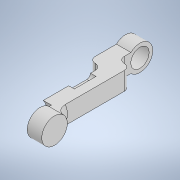
# Autodesk Inventor part: Рулевая тяга
Saved by Autodesk Inventor 2020 (Build 240168000, 168)
## iProperties
Created: 2021-07-18
Part Number: Рулевая тяга
Material: Типовые
Document SubType Name: Modeling
Designer: Антон
Density: 1 g/cm^3
Appearance: По умолчанию
Author: Антон
Autodesk Inventor part; units mm, degrees
ref_plane "YZ Plane" through (0, 0, 0) normal (1, 0, 0) x (0, 1, 0)
ref_plane "XZ Plane" through (0, 0, 0) normal (0, 1, 0) x (-1, 0, 0)
ref_plane "XY Plane" through (0, 0, 0) normal (0, 0, 1) x (1, 0, 0)
sketch "Эскиз1" plane through (0, 0, 0) normal (0, 1, 0) x (-1, 0, 0)
  line L0 (0, 0) -> (4, 0)
  line L1 (4, 0) -> (4, -23.1503)
  line L2 (4, -23.1503) -> (0, -23.1503)
  line L3 (0, -23.1503) -> (0, 0)
  line L4 (0, -23.1503) -> (7.35, -23.1503)
  line L5 (7.35, -23.1503) -> (7.35, -19.1503)
  line L6 (7.35, -19.1503) -> (0, -19.1503)
  line L7 (0, -19.1503) -> (0, -23.1503)
  line L8 (7.35, -19.1503) -> (3.35, -19.1503)
  line L9 (3.35, -19.1503) -> (3.35, -29.1503)
  line L10 (3.35, -29.1503) -> (7.35, -29.1503)
  line L11 (7.35, -29.1503) -> (7.35, -19.1503)
  line L12 (7.35, -23.1503) -> (4, -19.1503)
  line L13 (0, -19.1503) -> (3.35, -23.1503)
  point P0 (4, -19.1503)
  point P1 (0, -19.1503)
  point P2 (4, -19.1503)
  dimension "d10" = 4
  dimension "d11" = 7.35
  dimension "d36" = 29.1503
  dimension "d55" = 10
  constraints: 28 end point, 6 parallel, 4 point on line, 3 horizontal, 3 perpendicular, 2 equal length
  measures "d10" distance of L0.start L0.end
  measures "d11" distance between parallel lines of L3 L11
  measures "d36" distance between parallel lines of L10 L0
  measures "d55" distance of L10.end L5.end
extrude "Выдавливание1" add sketch "Эскиз1" along normal blind 5
fillet "Сопряжение2" radius 1.675 4 edges at (-4, 2.5, -19.1503) (-7.35, 2.5, -19.1503) (0, 2.5, -23.1503) (-3.35, 2.5, -23.1503)
sketch "Эскиз7" plane through (-7.35, 0, -29.1503) normal (-1, 0, 0) x (0, 0, 1)
  line L0 (0, 0) -> (0, 5) projected
  circle A0 centre (0, 2.5) radius 2.525
  circle A1 centre (0, 2.5) radius 3.525
  point P0 (29.1503, 0)
  point P1 (0, 4.975)
  point P2 (0, 0.025)
  dimension "d37" = 5.05
  dimension "d38" = 7.05
  constraints: 2 centre point, 1 coincident, 1 midpoint
  measures "d37" diameter of A0
  measures "d38" diameter of A1
extrude "Выдавливание5" add sketch "Эскиз7" against normal up to surface (4 mm away) contours A0 | A1
extrude "Выдавливание8" cut sketch "Эскиз7" against normal through all contours A0
sketch "Эскиз8" plane through (-4, 0, 0) normal (-1, 0, 0) x (0, 0, 1)
  line L0 (0, 0) -> (0, 5) projected
  circle A0 centre (0, 2.5) radius 2.525
  circle A1 centre (0, 2.5) radius 3.525
  point P0 (0, 4.975)
  point P1 (0, 0.025)
  dimension "d41" = 5.05
  dimension "d42" = 7.05
  constraints: 2 centre point, 1 coincident, 1 midpoint
  measures "d41" diameter of A0
  measures "d42" diameter of A1
extrude "Выдавливание6" add sketch "Эскиз8" against normal up to surface (4 mm away)
extrude "Выдавливание7" cut sketch "Эскиз8" against normal through all contours A0
sketch "Эскиз9" plane through (-4, 0, -21.4753) normal (1, 0, 0) x (0, 0, -1)
  arc A0 (-21.1209, 5) -> (-21.1209, 0) centre (-21.4753, 2.5) ccw projected
  circle A1 centre (-21.4753, 2.5) radius 4.025
  arc A2 (-18.9902, 5) -> (-18.9902, 0) centre (-21.4753, 2.5) ccw projected
  point P0 (-21.4753, 0)
  dimension "d61" = 0.5
  constraints: 1 centre point, 1 coincident
  measures "d61" radial gap between concentric circles of A1 A2
extrude "Выдавливание9" cut sketch "Эскиз9" along normal blind 2.25
sketch "Эскиз12" plane through (0, 0, -21.4753) normal (1, 0, 0) x (0, 0, -1)
  arc A0 (-18.9902, 5) -> (-18.9902, 0) centre (-21.4753, 2.5) ccw projected
  circle A1 centre (-21.4753, 2.5) radius 3.525
  circle A2 centre (-21.4753, 2.5) radius 2.525 projected
  circle A3 centre (-21.4753, 2.5) radius 2.525 projected
  circle A4 centre (-21.4753, 2.5) radius 2.525
  point P0 (-21.4753, 0)
  point P1 (-18.9902, 0)
  point P2 (-21.1209, 5)
  point P3 (-21.1209, 0)
  constraints: 2 coincident, 1 centre point, 3 other
extrude "Выдавливание12" add sketch "Эскиз12" along normal blind 2.25 contours A1 A0 | A2
fillet "Сопряжение6" radius 2.25 1 edges at (0, 2.5, -3.525)
sketch "Эскиз11" plane through (-4, 0, -17.4753) normal (-1, 0, 0) x (0, 0, 1)
  line L0 (6.3209, 5) -> (2.3209, 5) construction
  line L1 (6.3209, 6) -> (2.3209, 6)
  line L2 (2.3209, 4) -> (6.3209, 4)
  arc A0 (6.3209, 4) -> (6.3209, 6) centre (6.3209, 5) ccw
  arc A1 (2.3209, 6) -> (2.3209, 4) centre (2.3209, 5) ccw
  line L3 (0, 5) -> (14.3209, 5) projected
  point P0 (17.4753, 0)
  point P1 (4.3209, 5)
  dimension "d56" = 2
  dimension "d57" = 2
  dimension "d58" = 10
  constraints: 8 end point, 4 point on circle, 4 tangent, 2 centre point, 1 collinear, 1 horizontal, 1 midpoint, 1 parallel
  measures "d56" distance of point (4.321, 5) L0.end
  measures "d57" diameter of A1
  measures "d58" distance of L3.end point (4.321, 5)
extrude "Выдавливание11" cut sketch "Эскиз11" against normal blind 1.55
